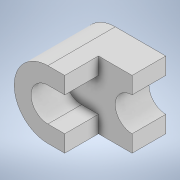
# Autodesk Inventor part: 件29
Saved by Autodesk Inventor 2020 (Build 240168000, 168)
## iProperties
Created: 2020-10-30
Part Number: 件29
Material: 一般
Document SubType Name: Modeling
Designer: USER
Density: 1 g/cm^3
Appearance: 預設
Author: USER
Autodesk Inventor part; units mm, degrees
ref_plane "YZ Plane" through (0, 0, 0) normal (1, 0, 0) x (0, 1, 0)
ref_plane "XZ Plane" through (0, 0, 0) normal (0, 1, 0) x (-1, 0, 0)
ref_plane "XY Plane" through (0, 0, 0) normal (0, 0, 1) x (1, 0, 0)
sketch "草圖1" plane through (0, 0, 0) normal (0, 0, 1) x (1, 0, 0)
  line L0 (25, -20) -> (-5, -20)
  line L1 (-25, 0) -> (-25, 0)
  line L2 (-5, 20) -> (25, 20)
  line L3 (25, -20) -> (-25, 20) construction
  line L4 (-25, -20) -> (25, 20) construction
  arc A0 (25, 10) -> (25, -10) centre (25, 0) ccw
  line L5 (25, 20) -> (25, 10)
  line L6 (25, -10) -> (25, -20)
  arc A1 (-5, 20) -> (-25, 0) centre (-5, 0) ccw
  arc A2 (-25, 0) -> (-5, -20) centre (-5, 0) ccw
  point P0 (0, 0)
  point P1 (-25, 0)
  dimension "d1" = 40
  dimension "d2" = 20
  dimension "d3" = 20
  constraints: 14 end point, 6 point on circle, 4 point on line, 4 tangent, 3 centre point, 3 parallel, 2 midpoint, 1 concentric, 1 horizontal, 1 perpendicular
  measures "d1" distance between parallel lines of L0 L2
  measures "d2" diameter of A0
  measures "d3" radius of A1
extrude "擠出1" add sketch "草圖1" along normal blind 20
sketch "草圖2" plane through (0, 0, 20) normal (0, 0, 1) x (1, 0, 0)
  arc A0 (-5, 20) -> (-5, -20) centre (-5, 0) ccw projected
  line L0 (25, 20) -> (-5, 20) projected
  line L1 (-5, 20) -> (5, 20)
  arc A1 (-5, 10) -> (-5, -10) centre (-5, 0) ccw
  arc A2 (-5, 20) -> (-5, -20) centre (-5, 0) ccw
  line L2 (5, 20) -> (5, 10)
  line L3 (5, 10) -> (-5, 10)
  line L4 (-5, 0) -> (21.3475, 0)
  line L5 (25, -20) -> (-5, -20)
  line L6 (5, -20) -> (5, -10)
  line L7 (5, -10) -> (-5, -10)
  point P0 (0, 0)
  dimension "d6" = 20
  dimension "d7" = 10
  constraints: 16 end point, 4 point on circle, 4 symmetric about line, 3 point on line, 2 centre point, 2 coincident, 2 tangent, 1 horizontal, 1 vertical
  measures "d6" diameter of A1
  measures "d7" distance of L1.end L0.end
extrude "擠出2" add sketch "草圖2" along normal blind 20
